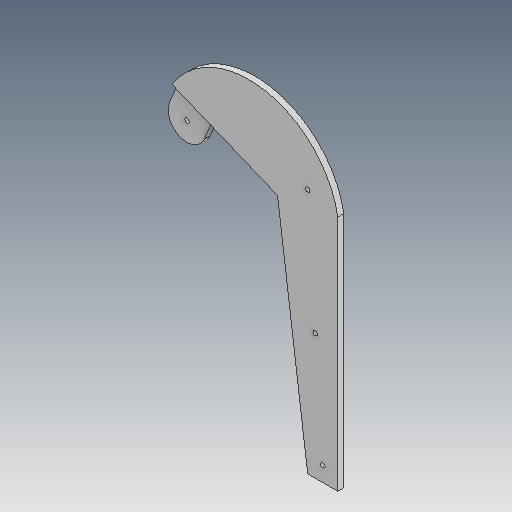
# Autodesk Inventor part: Halterung hinten oben
Saved by Autodesk Inventor 2020 (Build 240168000, 168)
## iProperties
Created: 2021-06-30
Part Number: Halterung hinten oben
Material: Generisch
Document SubType Name: Modeling
Designer: mike8
Density: 1 g/cm^3
Appearance: Vorgabe
Author: mike8
Autodesk Inventor part; units mm, degrees
ref_plane "YZ Plane" through (0, 0, 0) normal (1, 0, 0) x (0, 1, 0)
ref_plane "XZ Plane" through (0, 0, 0) normal (0, 1, 0) x (-1, 0, 0)
ref_plane "XY Plane" through (0, 0, 0) normal (0, 0, 1) x (1, 0, 0)
sketch "Skizze1" plane through (0, 0, 0) normal (0, 0, 1) x (1, 0, 0)
  line L0 (-103.8791, 0) -> (60.3442, 0) projected
  line L1 (0, -106.7819) -> (0, 196.5471) projected
  line L2 (29.5814, -63.4492) -> (29.5814, 94.1623)
  arc A0 (29.5814, 94.1623) -> (-80.4186, 115.4104) centre (-29.4958, 83.6793) ccw
  line L3 (-80.4186, 115.4104) -> (-10.4186, 86.5508)
  line L4 (-10.4186, 86.5508) -> (9.5814, -63.4492)
  line L5 (9.5814, -63.4492) -> (29.5814, -63.4492)
  point P0 (0, 0)
  point P1 (-57.3059, 105.8815)
  dimension "d0" = 120
  dimension "d2" = 20
  dimension "d3" = 40
  dimension "d4" = 120
  dimension "d6" = 150
  dimension "d24" = 70
  constraints: 8 end point, 2 point on circle, 1 centre point, 1 horizontal, 1 point on line, 1 vertical
  measures "d0" diameter of A0
  measures "d2" distance of L4.end L2.start
  measures "d3" distance from line of L2 L3.end
  measures "d4" angle of L4 L3
  measures "d6" vertical distance of L3.end L4.end
  measures "d24" horizontal distance of L3.start L3.end
extrude "Extrusion1" add sketch "Skizze1" along normal blind 4 contours L4 L1 A0 L2 L0 | L0 L2 L5 L4 | L4 L3 A0 L1
sketch "Skizze2" plane through (0, 0, 4) normal (0, 0, 1) x (1, 0, 0)
  arc A0 (-82.3244, 110.7879) -> (-59.2117, 101.2589) centre (-70.768, 106.0234) ccw projected
  line L0 (29.5814, -63.4492) -> (29.5814, 94.1623) projected
  line L1 (9.5814, -63.4492) -> (29.5814, -63.4492) projected
  point P0 (0, 0)
  point P1 (19.5814, -53.4492)
  dimension "d15" = 10
  dimension "d16" = 10
  measures "d15" distance from line of L0 point (19.581, -53.449)
  measures "d16" distance from line of L1 point (19.581, -53.449)
hole "Bohrung1" at (19.5814, -53.4492, 4) direction (0, 0, -1) diameter 3 end through all
sketch "Skizze3" plane through (-10.4186, 86.5508, 0) normal (-0.3811568, -0.9245104, 0) x (0.9245104, -0.3811568, 0)
  line L0 (34.0793, 4) -> (-75.7158, 4) projected
  line L1 (-75.7158, 4) -> (-50.7158, 4)
  line L2 (-50.7158, 4) -> (-50.7158, -11)
  line L3 (-50.7158, -11) -> (-75.7158, -11)
  line L4 (-75.7158, -11) -> (-75.7158, 4)
  point P0 (42.6216, 0)
  dimension "d25" = 15
  dimension "d26" = 25
  constraints: 8 end point, 2 parallel, 1 horizontal, 1 perpendicular
  measures "d25" distance of L3.end L0.end
  measures "d26" distance between parallel lines of L4 L2
extrude "Extrusion2" add sketch "Skizze3" along normal blind 10
sketch "Skizze4" plane through (-80.4186, 115.4104, -11) normal (-0.9245104, 0.3811568, 0) x (0, 0, 1)
  line L0 (11, 0) -> (11, 50.0739) projected
  line L1 (0, 0) -> (0, -10) projected
  line L2 (11, 0) -> (0, 0) projected
  line L3 (11, 0) -> (15, 0) projected
  line L4 (0, -10) -> (15, -10) projected
  line L5 (11, 0) -> (6, -5)
  line L6 (15, 0) -> (15, -10) projected
  line L7 (15, 0) -> (10, -5)
  line L8 (6, -5) -> (10, -5)
  point P0 (11, -76.046)
  point P1 (11, 22.2831)
  dimension "d30" = 5
  dimension "d31" = 5
  dimension "d32" = 45
  constraints: 6 end point, 1 parallel
  measures "d30" horizontal distance of L0.start L5.end
  measures "d31" horizontal distance of L3.end L7.end
  measures "d32" angle of L2 L5
extrude "Extrusion3" cut sketch "Skizze4" against normal blind 25 contours L2 L5 L8 L7 L6 L4 L1
sketch "Skizze5" plane through (-82.3244, 110.7879, -5) normal (-0.3811568, -0.9245104, 0) x (0.9245104, -0.3811568, 0)
  point P0 (118.3373, 5)
sketch "Skizze6" plane through (-82.3244, 110.7879, -5) normal (-0.3811568, -0.9245104, 0) x (0.9245104, -0.3811568, 0)
  point P0 (118.3373, 5)
sketch "Skizze7" plane through (-82.3244, 110.7879, -5) normal (-0.3811568, -0.9245104, 0) x (0.9245104, -0.3811568, 0)
  point P0 (118.3373, 5)
sketch "Skizze8" plane through (-82.3244, 110.7879, -5) normal (-0.3811568, -0.9245104, 0) x (0.9245104, -0.3811568, 0)
  line L0 (25, 4) -> (25, 0) projected
  line L1 (0, 0) -> (25, 0)
  line L2 (25, 0) -> (25, 4)
  line L3 (25, 4) -> (0, 4)
  line L4 (0, 4) -> (0, 0)
  point P0 (118.3373, 5)
  point P1 (25, 0)
  constraints: 8 end point, 2 parallel, 1 horizontal, 1 perpendicular
extrude "Extrusion4" add sketch "Skizze8" along normal blind 25
sketch "Skizze9" plane through (-91.8533, 87.6751, -1) normal (0, 0, 1) x (0.9245104, -0.3811568, 0)
  arc A0 (0, 12.5) -> (25, 12.5) centre (12.5, 12.5) ccw
  line L0 (0, 25) -> (0, 0) projected
  line L1 (25, 0) -> (0, 0) projected
  line L2 (25, 25) -> (25, 0) projected
  line L3 (25, 12.5) -> (25, 0)
  line L4 (0, 0) -> (0, 12.5)
  point P0 (118.3373, -46.046)
  point P1 (12.5, 0)
  dimension "d37" = 25
  dimension "d38" = 12.5
  constraints: 4 end point, 2 midpoint, 2 point on circle, 2 tangent, 1 centre point, 1 parallel, 1 vertical
  measures "d37" diameter of A0
  measures "d38" distance from line of L1 A0.centre
extrude "Extrusion5" cut sketch "Skizze9" against normal blind 30
sketch "Skizze10" plane through (-82.3244, 110.7879, -1) normal (0, 0, 1) x (0.9245104, -0.3811568, 0)
  arc A0 (0, -12.5) -> (25, -12.5) centre (12.5, -12.5) ccw projected
  point P0 (118.3373, -71.046)
  point P1 (12.5, -12.5)
  dimension "d41" = 0
  dimension "d42" = 0
  measures "d41" distance of A0.centre point (12.5, -12.5)
  measures "d42" distance of A0.centre point (12.5, -12.5)
hole "Bohrung2" at (-75.5325, 94.467, -1) direction (0, 0, -1) diameter 3 end through all
sketch "Skizze12" plane through (0, 0, 4) normal (0, 0, 1) x (1, 0, 0)
  line L0 (-57.3059, 105.8815) -> (-10.4186, 86.5508) projected
  line L1 (29.5814, -63.4492) -> (29.5814, 94.1623) projected
  point P0 (0, 0)
  point P1 (9.5814, 99.9383)
  point P2 (14.5814, 19.9383)
  dimension "d63" = 20
  dimension "d64" = 20
  dimension "d65" = 80
  dimension "d66" = 15
  measures "d63" distance from line of L0 point (9.581, 99.938)
  measures "d64" distance from line of L1 point (9.581, 99.938)
  measures "d65" vertical distance of point (14.581, 19.938) point (9.581, 99.938)
  measures "d66" distance from line of L1 point (14.581, 19.938)
hole "Bohrung4" at (9.5814, 99.9383, 4) at (14.5814, 19.9383, 4) direction (0, 0, -1) diameter 3 end through all
